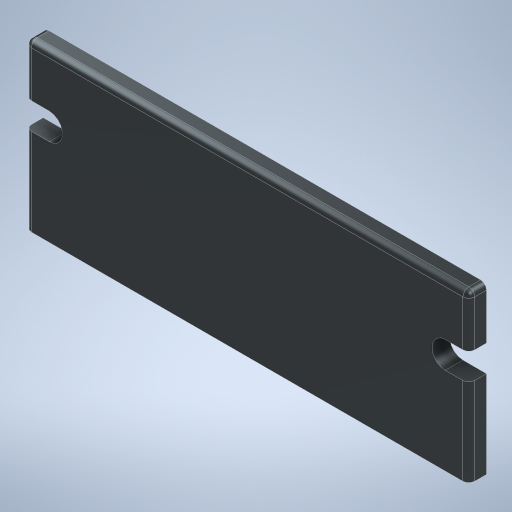
# Autodesk Inventor part: MirrorControllerModel
Saved by Autodesk Inventor 2023 (Build 270158000, 158)
## iProperties
Created: 2022-10-22
Part Number: MirrorControllerModel
Material: Iron, Cast
Document SubType Name: Modeling
Designer: Miner
Density: 7.15 g/cm^3
Appearance: Iron Gray
Author: Miner
Autodesk Inventor part; units mm, degrees
ref_plane "YZ Plane" through (0, 0, 0) normal (1, 0, 0) x (0, 1, 0)
ref_plane "XZ Plane" through (0, 0, 0) normal (0, 1, 0) x (-1, 0, 0)
ref_plane "XY Plane" through (0, 0, 0) normal (0, 0, 1) x (1, 0, 0)
sketch "Sketch1" plane through (0, 0, 0) normal (0, 0, 1) x (1, 0, 0)
  line L0 (0, 0) -> (-75, 0)
  line L1 (-75, 28) -> (0, 28)
  line L2 (0, 28) -> (0, 19.25) construction
  line L3 (0, 17) -> (-75, 17) construction
  line L4 (0, 17) -> (-4, 17) construction
  arc A0 (-4, 19.25) -> (-4, 14.75) centre (-4, 17) ccw
  line L5 (-4, 19.25) -> (0, 19.25)
  line L6 (-4, 14.75) -> (0, 14.75)
  line L7 (0, 28) -> (0, 19.25)
  line L8 (0, 14.75) -> (0, 0)
  line L9 (-37.5, 28) -> (-37.5, 0) construction
  arc A1 (-71, 14.75) -> (-71, 19.25) centre (-71, 17) ccw
  line L10 (-71, 19.25) -> (-75, 19.25)
  line L11 (-71, 14.75) -> (-75, 14.75)
  line L12 (-75, 0) -> (-75, 14.75)
  line L13 (-75, 19.25) -> (-75, 28)
  dimension "d0" = 75
  dimension "d1" = 28
  dimension "d2" = 11
  dimension "d3" = 4
  dimension "d4" = 4.5
  constraints: 28 end point, 8 perpendicular, 5 parallel, 5 symmetric about line, 4 point on circle, 2 centre point, 2 midpoint, 2 tangent, 1 coincident, 1 horizontal, 1 point on line, 1 other
  measures "d0" distance of L1.start L1.end
  measures "d1" distance of L0.end L1.start
  measures "d2" distance of L1.end L3.start
  measures "d3" distance of L3.start L4.end
  measures "d4" diameter of A0
extrude "Extrusion1" add sketch "Sketch1" along normal blind 3
fillet "Fillet1" radius 1 7 edges at (-37.5, 28, 3) (0, 28, 1.5) (-75, 28, 1.5) (0, 23.625, 3) (0, 7.375, 3) (-75, 23.625, 3) (-75, 7.375, 3)
body "Solid1"
